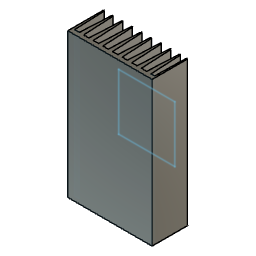
Heat Sink Uncut v1 (Autodesk Fusion 360 design; units mm, degrees)
Autodesk Fusion 360 part; units mm, degrees
sketch "Sketch1" plane through (0, 0, 0) normal (0, 0, 1) x (1, 0, 0)
  line L0 (0, 0) -> (105.15, 0)
  spline S0 degree 5 poles (10.96, 44) (10.99, 44.0758) (11.05, 44.2209) (11.14, 44.4187) (11.26, 44.6419) (11.41, 44.8491) (11.56, 44.9779) (11.71, 45.022) (11.86, 44.9779) (12.01, 44.8491) (12.16, 44.6419) (12.28, 44.4187) (12.37, 44.2209) (12.43, 44.0758) (12.46, 44) knots 0 0 0 0 0 0 0.1 0.2 0.3 0.4 0.5 0.6 0.7 0.8 0.9 1 1 1 1 1 1
  line L1 (10.96, 44) -> (9, 5.4)
  line L2 (12.46, 44) -> (14.42, 5.4)
  spline S1 degree 5 poles (10.96, 44) (10.99, 44.0758) (11.05, 44.2209) (11.14, 44.4187) (11.26, 44.6419) (11.41, 44.8491) (11.56, 44.9779) (11.71, 45.022) (11.86, 44.9779) (12.01, 44.8491) (12.16, 44.6419) (12.28, 44.4187) (12.37, 44.2209) (12.43, 44.0758) (12.46, 44) knots 0 0 0 0 0 0 0.1 0.2 0.3 0.4 0.5 0.6 0.7 0.8 0.9 1 1 1 1 1 1
  line L3 (10.96, 44) -> (9, 5.4)
  line L4 (12.46, 44) -> (14.42, 5.4)
  spline S2 degree 5 poles (10.96, 44) (10.99, 44.0758) (11.05, 44.2209) (11.14, 44.4187) (11.26, 44.6419) (11.41, 44.8491) (11.56, 44.9779) (11.71, 45.022) (11.86, 44.9779) (12.01, 44.8491) (12.16, 44.6419) (12.28, 44.4187) (12.37, 44.2209) (12.43, 44.0758) (12.46, 44) knots 0 0 0 0 0 0 0.1 0.2 0.3 0.4 0.5 0.6 0.7 0.8 0.9 1 1 1 1 1 1
  spline S3 degree 5 poles (10.96, 44) (10.99, 44.0758) (11.05, 44.2209) (11.14, 44.4187) (11.26, 44.6419) (11.41, 44.8491) (11.56, 44.9779) (11.71, 45.022) (11.86, 44.9779) (12.01, 44.8491) (12.16, 44.6419) (12.28, 44.4187) (12.37, 44.2209) (12.43, 44.0758) (12.46, 44) knots 0 0 0 0 0 0 0.1 0.2 0.3 0.4 0.5 0.6 0.7 0.8 0.9 1 1 1 1 1 1
  line L5 (10.96, 44) -> (9, 5.4)
  line L6 (12.46, 44) -> (14.42, 5.4)
  spline S4 degree 5 poles (10.96, 44) (10.99, 44.0758) (11.05, 44.2209) (11.14, 44.4187) (11.26, 44.6419) (11.41, 44.8491) (11.56, 44.9779) (11.71, 45.022) (11.86, 44.9779) (12.01, 44.8491) (12.16, 44.6419) (12.28, 44.4187) (12.37, 44.2209) (12.43, 44.0758) (12.46, 44) knots 0 0 0 0 0 0 0.1 0.2 0.3 0.4 0.5 0.6 0.7 0.8 0.9 1 1 1 1 1 1
  spline S5 degree 5 poles (10.96, 44) (10.99, 44.0758) (11.05, 44.2209) (11.14, 44.4187) (11.26, 44.6419) (11.41, 44.8491) (11.56, 44.9779) (11.71, 45.022) (11.86, 44.9779) (12.01, 44.8491) (12.16, 44.6419) (12.28, 44.4187) (12.37, 44.2209) (12.43, 44.0758) (12.46, 44) knots 0 0 0 0 0 0 0.1 0.2 0.3 0.4 0.5 0.6 0.7 0.8 0.9 1 1 1 1 1 1
  spline S6 degree 5 poles (10.96, 44) (10.99, 44.0758) (11.05, 44.2209) (11.14, 44.4187) (11.26, 44.6419) (11.41, 44.8491) (11.56, 44.9779) (11.71, 45.022) (11.86, 44.9779) (12.01, 44.8491) (12.16, 44.6419) (12.28, 44.4187) (12.37, 44.2209) (12.43, 44.0758) (12.46, 44) knots 0 0 0 0 0 0 0.1 0.2 0.3 0.4 0.5 0.6 0.7 0.8 0.9 1 1 1 1 1 1
  spline S7 degree 5 poles (10.96, 44) (10.99, 44.0758) (11.05, 44.2209) (11.14, 44.4187) (11.26, 44.6419) (11.41, 44.8491) (11.56, 44.9779) (11.71, 45.022) (11.86, 44.9779) (12.01, 44.8491) (12.16, 44.6419) (12.28, 44.4187) (12.37, 44.2209) (12.43, 44.0758) (12.46, 44) knots 0 0 0 0 0 0 0.1 0.2 0.3 0.4 0.5 0.6 0.7 0.8 0.9 1 1 1 1 1 1
  line L7 (10.96, 44) -> (9, 5.4)
  line L8 (12.46, 44) -> (14.42, 5.4)
  spline S8 degree 5 poles (22.96, 44) (22.99, 44.0758) (23.05, 44.2209) (23.14, 44.4187) (23.26, 44.6419) (23.41, 44.8491) (23.56, 44.9779) (23.71, 45.022) (23.86, 44.9779) (24.01, 44.8491) (24.16, 44.6419) (24.28, 44.4187) (24.37, 44.2209) (24.43, 44.0758) (24.46, 44) knots 0 0 0 0 0 0 0.1 0.2 0.3 0.4 0.5 0.6 0.7 0.8 0.9 1 1 1 1 1 1
  spline S9 degree 5 poles (22.96, 44) (22.99, 44.0758) (23.05, 44.2209) (23.14, 44.4187) (23.26, 44.6419) (23.41, 44.8491) (23.56, 44.9779) (23.71, 45.022) (23.86, 44.9779) (24.01, 44.8491) (24.16, 44.6419) (24.28, 44.4187) (24.37, 44.2209) (24.43, 44.0758) (24.46, 44) knots 0 0 0 0 0 0 0.1 0.2 0.3 0.4 0.5 0.6 0.7 0.8 0.9 1 1 1 1 1 1
  spline S10 degree 5 poles (22.96, 44) (22.99, 44.0758) (23.05, 44.2209) (23.14, 44.4187) (23.26, 44.6419) (23.41, 44.8491) (23.56, 44.9779) (23.71, 45.022) (23.86, 44.9779) (24.01, 44.8491) (24.16, 44.6419) (24.28, 44.4187) (24.37, 44.2209) (24.43, 44.0758) (24.46, 44) knots 0 0 0 0 0 0 0.1 0.2 0.3 0.4 0.5 0.6 0.7 0.8 0.9 1 1 1 1 1 1
  spline S11 degree 5 poles (22.96, 44) (22.99, 44.0758) (23.05, 44.2209) (23.14, 44.4187) (23.26, 44.6419) (23.41, 44.8491) (23.56, 44.9779) (23.71, 45.022) (23.86, 44.9779) (24.01, 44.8491) (24.16, 44.6419) (24.28, 44.4187) (24.37, 44.2209) (24.43, 44.0758) (24.46, 44) knots 0 0 0 0 0 0 0.1 0.2 0.3 0.4 0.5 0.6 0.7 0.8 0.9 1 1 1 1 1 1
  spline S12 degree 5 poles (22.96, 44) (22.99, 44.0758) (23.05, 44.2209) (23.14, 44.4187) (23.26, 44.6419) (23.41, 44.8491) (23.56, 44.9779) (23.71, 45.022) (23.86, 44.9779) (24.01, 44.8491) (24.16, 44.6419) (24.28, 44.4187) (24.37, 44.2209) (24.43, 44.0758) (24.46, 44) knots 0 0 0 0 0 0 0.1 0.2 0.3 0.4 0.5 0.6 0.7 0.8 0.9 1 1 1 1 1 1
  spline S13 degree 5 poles (22.96, 44) (22.99, 44.0758) (23.05, 44.2209) (23.14, 44.4187) (23.26, 44.6419) (23.41, 44.8491) (23.56, 44.9779) (23.71, 45.022) (23.86, 44.9779) (24.01, 44.8491) (24.16, 44.6419) (24.28, 44.4187) (24.37, 44.2209) (24.43, 44.0758) (24.46, 44) knots 0 0 0 0 0 0 0.1 0.2 0.3 0.4 0.5 0.6 0.7 0.8 0.9 1 1 1 1 1 1
  spline S14 degree 5 poles (22.96, 44) (22.99, 44.0758) (23.05, 44.2209) (23.14, 44.4187) (23.26, 44.6419) (23.41, 44.8491) (23.56, 44.9779) (23.71, 45.022) (23.86, 44.9779) (24.01, 44.8491) (24.16, 44.6419) (24.28, 44.4187) (24.37, 44.2209) (24.43, 44.0758) (24.46, 44) knots 0 0 0 0 0 0 0.1 0.2 0.3 0.4 0.5 0.6 0.7 0.8 0.9 1 1 1 1 1 1
  spline S15 degree 5 poles (22.96, 44) (22.99, 44.0758) (23.05, 44.2209) (23.14, 44.4187) (23.26, 44.6419) (23.41, 44.8491) (23.56, 44.9779) (23.71, 45.022) (23.86, 44.9779) (24.01, 44.8491) (24.16, 44.6419) (24.28, 44.4187) (24.37, 44.2209) (24.43, 44.0758) (24.46, 44) knots 0 0 0 0 0 0 0.1 0.2 0.3 0.4 0.5 0.6 0.7 0.8 0.9 1 1 1 1 1 1
  line L9 (22.96, 44) -> (21, 5.4)
  line L10 (24.46, 44) -> (26.42, 5.4)
  spline S16 degree 5 poles (34.96, 44) (34.99, 44.0758) (35.05, 44.2209) (35.14, 44.4187) (35.26, 44.6419) (35.41, 44.8491) (35.56, 44.9779) (35.71, 45.022) (35.86, 44.9779) (36.01, 44.8491) (36.16, 44.6419) (36.28, 44.4187) (36.37, 44.2209) (36.43, 44.0758) (36.46, 44) knots 0 0 0 0 0 0 0.1 0.2 0.3 0.4 0.5 0.6 0.7 0.8 0.9 1 1 1 1 1 1
  spline S17 degree 5 poles (34.96, 44) (34.99, 44.0758) (35.05, 44.2209) (35.14, 44.4187) (35.26, 44.6419) (35.41, 44.8491) (35.56, 44.9779) (35.71, 45.022) (35.86, 44.9779) (36.01, 44.8491) (36.16, 44.6419) (36.28, 44.4187) (36.37, 44.2209) (36.43, 44.0758) (36.46, 44) knots 0 0 0 0 0 0 0.1 0.2 0.3 0.4 0.5 0.6 0.7 0.8 0.9 1 1 1 1 1 1
  spline S18 degree 5 poles (34.96, 44) (34.99, 44.0758) (35.05, 44.2209) (35.14, 44.4187) (35.26, 44.6419) (35.41, 44.8491) (35.56, 44.9779) (35.71, 45.022) (35.86, 44.9779) (36.01, 44.8491) (36.16, 44.6419) (36.28, 44.4187) (36.37, 44.2209) (36.43, 44.0758) (36.46, 44) knots 0 0 0 0 0 0 0.1 0.2 0.3 0.4 0.5 0.6 0.7 0.8 0.9 1 1 1 1 1 1
  spline S19 degree 5 poles (34.96, 44) (34.99, 44.0758) (35.05, 44.2209) (35.14, 44.4187) (35.26, 44.6419) (35.41, 44.8491) (35.56, 44.9779) (35.71, 45.022) (35.86, 44.9779) (36.01, 44.8491) (36.16, 44.6419) (36.28, 44.4187) (36.37, 44.2209) (36.43, 44.0758) (36.46, 44) knots 0 0 0 0 0 0 0.1 0.2 0.3 0.4 0.5 0.6 0.7 0.8 0.9 1 1 1 1 1 1
  spline S20 degree 5 poles (34.96, 44) (34.99, 44.0758) (35.05, 44.2209) (35.14, 44.4187) (35.26, 44.6419) (35.41, 44.8491) (35.56, 44.9779) (35.71, 45.022) (35.86, 44.9779) (36.01, 44.8491) (36.16, 44.6419) (36.28, 44.4187) (36.37, 44.2209) (36.43, 44.0758) (36.46, 44) knots 0 0 0 0 0 0 0.1 0.2 0.3 0.4 0.5 0.6 0.7 0.8 0.9 1 1 1 1 1 1
  spline S21 degree 5 poles (34.96, 44) (34.99, 44.0758) (35.05, 44.2209) (35.14, 44.4187) (35.26, 44.6419) (35.41, 44.8491) (35.56, 44.9779) (35.71, 45.022) (35.86, 44.9779) (36.01, 44.8491) (36.16, 44.6419) (36.28, 44.4187) (36.37, 44.2209) (36.43, 44.0758) (36.46, 44) knots 0 0 0 0 0 0 0.1 0.2 0.3 0.4 0.5 0.6 0.7 0.8 0.9 1 1 1 1 1 1
  spline S22 degree 5 poles (34.96, 44) (34.99, 44.0758) (35.05, 44.2209) (35.14, 44.4187) (35.26, 44.6419) (35.41, 44.8491) (35.56, 44.9779) (35.71, 45.022) (35.86, 44.9779) (36.01, 44.8491) (36.16, 44.6419) (36.28, 44.4187) (36.37, 44.2209) (36.43, 44.0758) (36.46, 44) knots 0 0 0 0 0 0 0.1 0.2 0.3 0.4 0.5 0.6 0.7 0.8 0.9 1 1 1 1 1 1
  spline S23 degree 5 poles (34.96, 44) (34.99, 44.0758) (35.05, 44.2209) (35.14, 44.4187) (35.26, 44.6419) (35.41, 44.8491) (35.56, 44.9779) (35.71, 45.022) (35.86, 44.9779) (36.01, 44.8491) (36.16, 44.6419) (36.28, 44.4187) (36.37, 44.2209) (36.43, 44.0758) (36.46, 44) knots 0 0 0 0 0 0 0.1 0.2 0.3 0.4 0.5 0.6 0.7 0.8 0.9 1 1 1 1 1 1
  line L11 (34.96, 44) -> (33, 5.4)
  line L12 (36.46, 44) -> (38.42, 5.4)
  spline S24 degree 5 poles (46.96, 44) (46.99, 44.0758) (47.05, 44.2209) (47.14, 44.4187) (47.26, 44.6419) (47.41, 44.8491) (47.56, 44.9779) (47.71, 45.022) (47.86, 44.9779) (48.01, 44.8491) (48.16, 44.6419) (48.28, 44.4187) (48.37, 44.2209) (48.43, 44.0758) (48.46, 44) knots 0 0 0 0 0 0 0.1 0.2 0.3 0.4 0.5 0.6 0.7 0.8 0.9 1 1 1 1 1 1
  spline S25 degree 5 poles (46.96, 44) (46.99, 44.0758) (47.05, 44.2209) (47.14, 44.4187) (47.26, 44.6419) (47.41, 44.8491) (47.56, 44.9779) (47.71, 45.022) (47.86, 44.9779) (48.01, 44.8491) (48.16, 44.6419) (48.28, 44.4187) (48.37, 44.2209) (48.43, 44.0758) (48.46, 44) knots 0 0 0 0 0 0 0.1 0.2 0.3 0.4 0.5 0.6 0.7 0.8 0.9 1 1 1 1 1 1
  spline S26 degree 5 poles (46.96, 44) (46.99, 44.0758) (47.05, 44.2209) (47.14, 44.4187) (47.26, 44.6419) (47.41, 44.8491) (47.56, 44.9779) (47.71, 45.022) (47.86, 44.9779) (48.01, 44.8491) (48.16, 44.6419) (48.28, 44.4187) (48.37, 44.2209) (48.43, 44.0758) (48.46, 44) knots 0 0 0 0 0 0 0.1 0.2 0.3 0.4 0.5 0.6 0.7 0.8 0.9 1 1 1 1 1 1
  spline S27 degree 5 poles (46.96, 44) (46.99, 44.0758) (47.05, 44.2209) (47.14, 44.4187) (47.26, 44.6419) (47.41, 44.8491) (47.56, 44.9779) (47.71, 45.022) (47.86, 44.9779) (48.01, 44.8491) (48.16, 44.6419) (48.28, 44.4187) (48.37, 44.2209) (48.43, 44.0758) (48.46, 44) knots 0 0 0 0 0 0 0.1 0.2 0.3 0.4 0.5 0.6 0.7 0.8 0.9 1 1 1 1 1 1
  spline S28 degree 5 poles (46.96, 44) (46.99, 44.0758) (47.05, 44.2209) (47.14, 44.4187) (47.26, 44.6419) (47.41, 44.8491) (47.56, 44.9779) (47.71, 45.022) (47.86, 44.9779) (48.01, 44.8491) (48.16, 44.6419) (48.28, 44.4187) (48.37, 44.2209) (48.43, 44.0758) (48.46, 44) knots 0 0 0 0 0 0 0.1 0.2 0.3 0.4 0.5 0.6 0.7 0.8 0.9 1 1 1 1 1 1
  spline S29 degree 5 poles (46.96, 44) (46.99, 44.0758) (47.05, 44.2209) (47.14, 44.4187) (47.26, 44.6419) (47.41, 44.8491) (47.56, 44.9779) (47.71, 45.022) (47.86, 44.9779) (48.01, 44.8491) (48.16, 44.6419) (48.28, 44.4187) (48.37, 44.2209) (48.43, 44.0758) (48.46, 44) knots 0 0 0 0 0 0 0.1 0.2 0.3 0.4 0.5 0.6 0.7 0.8 0.9 1 1 1 1 1 1
  spline S30 degree 5 poles (46.96, 44) (46.99, 44.0758) (47.05, 44.2209) (47.14, 44.4187) (47.26, 44.6419) (47.41, 44.8491) (47.56, 44.9779) (47.71, 45.022) (47.86, 44.9779) (48.01, 44.8491) (48.16, 44.6419) (48.28, 44.4187) (48.37, 44.2209) (48.43, 44.0758) (48.46, 44) knots 0 0 0 0 0 0 0.1 0.2 0.3 0.4 0.5 0.6 0.7 0.8 0.9 1 1 1 1 1 1
  spline S31 degree 5 poles (46.96, 44) (46.99, 44.0758) (47.05, 44.2209) (47.14, 44.4187) (47.26, 44.6419) (47.41, 44.8491) (47.56, 44.9779) (47.71, 45.022) (47.86, 44.9779) (48.01, 44.8491) (48.16, 44.6419) (48.28, 44.4187) (48.37, 44.2209) (48.43, 44.0758) (48.46, 44) knots 0 0 0 0 0 0 0.1 0.2 0.3 0.4 0.5 0.6 0.7 0.8 0.9 1 1 1 1 1 1
  line L13 (46.96, 44) -> (45, 5.4)
  line L14 (48.46, 44) -> (50.42, 5.4)
  spline S32 degree 5 poles (58.96, 44) (58.99, 44.0758) (59.05, 44.2209) (59.14, 44.4187) (59.26, 44.6419) (59.41, 44.8491) (59.56, 44.9779) (59.71, 45.022) (59.86, 44.9779) (60.01, 44.8491) (60.16, 44.6419) (60.28, 44.4187) (60.37, 44.2209) (60.43, 44.0758) (60.46, 44) knots 0 0 0 0 0 0 0.1 0.2 0.3 0.4 0.5 0.6 0.7 0.8 0.9 1 1 1 1 1 1
  spline S33 degree 5 poles (58.96, 44) (58.99, 44.0758) (59.05, 44.2209) (59.14, 44.4187) (59.26, 44.6419) (59.41, 44.8491) (59.56, 44.9779) (59.71, 45.022) (59.86, 44.9779) (60.01, 44.8491) (60.16, 44.6419) (60.28, 44.4187) (60.37, 44.2209) (60.43, 44.0758) (60.46, 44) knots 0 0 0 0 0 0 0.1 0.2 0.3 0.4 0.5 0.6 0.7 0.8 0.9 1 1 1 1 1 1
  spline S34 degree 5 poles (58.96, 44) (58.99, 44.0758) (59.05, 44.2209) (59.14, 44.4187) (59.26, 44.6419) (59.41, 44.8491) (59.56, 44.9779) (59.71, 45.022) (59.86, 44.9779) (60.01, 44.8491) (60.16, 44.6419) (60.28, 44.4187) (60.37, 44.2209) (60.43, 44.0758) (60.46, 44) knots 0 0 0 0 0 0 0.1 0.2 0.3 0.4 0.5 0.6 0.7 0.8 0.9 1 1 1 1 1 1
  spline S35 degree 5 poles (58.96, 44) (58.99, 44.0758) (59.05, 44.2209) (59.14, 44.4187) (59.26, 44.6419) (59.41, 44.8491) (59.56, 44.9779) (59.71, 45.022) (59.86, 44.9779) (60.01, 44.8491) (60.16, 44.6419) (60.28, 44.4187) (60.37, 44.2209) (60.43, 44.0758) (60.46, 44) knots 0 0 0 0 0 0 0.1 0.2 0.3 0.4 0.5 0.6 0.7 0.8 0.9 1 1 1 1 1 1
  spline S36 degree 5 poles (58.96, 44) (58.99, 44.0758) (59.05, 44.2209) (59.14, 44.4187) (59.26, 44.6419) (59.41, 44.8491) (59.56, 44.9779) (59.71, 45.022) (59.86, 44.9779) (60.01, 44.8491) (60.16, 44.6419) (60.28, 44.4187) (60.37, 44.2209) (60.43, 44.0758) (60.46, 44) knots 0 0 0 0 0 0 0.1 0.2 0.3 0.4 0.5 0.6 0.7 0.8 0.9 1 1 1 1 1 1
  spline S37 degree 5 poles (58.96, 44) (58.99, 44.0758) (59.05, 44.2209) (59.14, 44.4187) (59.26, 44.6419) (59.41, 44.8491) (59.56, 44.9779) (59.71, 45.022) (59.86, 44.9779) (60.01, 44.8491) (60.16, 44.6419) (60.28, 44.4187) (60.37, 44.2209) (60.43, 44.0758) (60.46, 44) knots 0 0 0 0 0 0 0.1 0.2 0.3 0.4 0.5 0.6 0.7 0.8 0.9 1 1 1 1 1 1
  spline S38 degree 5 poles (58.96, 44) (58.99, 44.0758) (59.05, 44.2209) (59.14, 44.4187) (59.26, 44.6419) (59.41, 44.8491) (59.56, 44.9779) (59.71, 45.022) (59.86, 44.9779) (60.01, 44.8491) (60.16, 44.6419) (60.28, 44.4187) (60.37, 44.2209) (60.43, 44.0758) (60.46, 44) knots 0 0 0 0 0 0 0.1 0.2 0.3 0.4 0.5 0.6 0.7 0.8 0.9 1 1 1 1 1 1
  spline S39 degree 5 poles (58.96, 44) (58.99, 44.0758) (59.05, 44.2209) (59.14, 44.4187) (59.26, 44.6419) (59.41, 44.8491) (59.56, 44.9779) (59.71, 45.022) (59.86, 44.9779) (60.01, 44.8491) (60.16, 44.6419) (60.28, 44.4187) (60.37, 44.2209) (60.43, 44.0758) (60.46, 44) knots 0 0 0 0 0 0 0.1 0.2 0.3 0.4 0.5 0.6 0.7 0.8 0.9 1 1 1 1 1 1
  line L15 (58.96, 44) -> (57, 5.4)
  line L16 (60.46, 44) -> (62.42, 5.4)
  spline S40 degree 5 poles (58.96, 44) (58.99, 44.0758) (59.05, 44.2209) (59.14, 44.4187) (59.26, 44.6419) (59.41, 44.8491) (59.56, 44.9779) (59.71, 45.022) (59.86, 44.9779) (60.01, 44.8491) (60.16, 44.6419) (60.28, 44.4187) (60.37, 44.2209) (60.43, 44.0758) (60.46, 44) knots 0 0 0 0 0 0 0.1 0.2 0.3 0.4 0.5 0.6 0.7 0.8 0.9 1 1 1 1 1 1
  spline S41 degree 5 poles (58.96, 44) (58.99, 44.0758) (59.05, 44.2209) (59.14, 44.4187) (59.26, 44.6419) (59.41, 44.8491) (59.56, 44.9779) (59.71, 45.022) (59.86, 44.9779) (60.01, 44.8491) (60.16, 44.6419) (60.28, 44.4187) (60.37, 44.2209) (60.43, 44.0758) (60.46, 44) knots 0 0 0 0 0 0 0.1 0.2 0.3 0.4 0.5 0.6 0.7 0.8 0.9 1 1 1 1 1 1
  spline S42 degree 5 poles (58.96, 44) (58.99, 44.0758) (59.05, 44.2209) (59.14, 44.4187) (59.26, 44.6419) (59.41, 44.8491) (59.56, 44.9779) (59.71, 45.022) (59.86, 44.9779) (60.01, 44.8491) (60.16, 44.6419) (60.28, 44.4187) (60.37, 44.2209) (60.43, 44.0758) (60.46, 44) knots 0 0 0 0 0 0 0.1 0.2 0.3 0.4 0.5 0.6 0.7 0.8 0.9 1 1 1 1 1 1
  spline S43 degree 5 poles (58.96, 44) (58.99, 44.0758) (59.05, 44.2209) (59.14, 44.4187) (59.26, 44.6419) (59.41, 44.8491) (59.56, 44.9779) (59.71, 45.022) (59.86, 44.9779) (60.01, 44.8491) (60.16, 44.6419) (60.28, 44.4187) (60.37, 44.2209) (60.43, 44.0758) (60.46, 44) knots 0 0 0 0 0 0 0.1 0.2 0.3 0.4 0.5 0.6 0.7 0.8 0.9 1 1 1 1 1 1
  spline S44 degree 5 poles (58.96, 44) (58.99, 44.0758) (59.05, 44.2209) (59.14, 44.4187) (59.26, 44.6419) (59.41, 44.8491) (59.56, 44.9779) (59.71, 45.022) (59.86, 44.9779) (60.01, 44.8491) (60.16, 44.6419) (60.28, 44.4187) (60.37, 44.2209) (60.43, 44.0758) (60.46, 44) knots 0 0 0 0 0 0 0.1 0.2 0.3 0.4 0.5 0.6 0.7 0.8 0.9 1 1 1 1 1 1
  spline S45 degree 5 poles (58.96, 44) (58.99, 44.0758) (59.05, 44.2209) (59.14, 44.4187) (59.26, 44.6419) (59.41, 44.8491) (59.56, 44.9779) (59.71, 45.022) (59.86, 44.9779) (60.01, 44.8491) (60.16, 44.6419) (60.28, 44.4187) (60.37, 44.2209) (60.43, 44.0758) (60.46, 44) knots 0 0 0 0 0 0 0.1 0.2 0.3 0.4 0.5 0.6 0.7 0.8 0.9 1 1 1 1 1 1
  spline S46 degree 5 poles (58.96, 44) (58.99, 44.0758) (59.05, 44.2209) (59.14, 44.4187) (59.26, 44.6419) (59.41, 44.8491) (59.56, 44.9779) (59.71, 45.022) (59.86, 44.9779) (60.01, 44.8491) (60.16, 44.6419) (60.28, 44.4187) (60.37, 44.2209) (60.43, 44.0758) (60.46, 44) knots 0 0 0 0 0 0 0.1 0.2 0.3 0.4 0.5 0.6 0.7 0.8 0.9 1 1 1 1 1 1
  spline S47 degree 5 poles (58.96, 44) (58.99, 44.0758) (59.05, 44.2209) (59.14, 44.4187) (59.26, 44.6419) (59.41, 44.8491) (59.56, 44.9779) (59.71, 45.022) (59.86, 44.9779) (60.01, 44.8491) (60.16, 44.6419) (60.28, 44.4187) (60.37, 44.2209) (60.43, 44.0758) (60.46, 44) knots 0 0 0 0 0 0 0.1 0.2 0.3 0.4 0.5 0.6 0.7 0.8 0.9 1 1 1 1 1 1
  spline S48 degree 5 poles (70.96, 44) (70.99, 44.0758) (71.05, 44.2209) (71.14, 44.4187) (71.26, 44.6419) (71.41, 44.8491) (71.56, 44.9779) (71.71, 45.022) (71.86, 44.9779) (72.01, 44.8491) (72.16, 44.6419) (72.28, 44.4187) (72.37, 44.2209) (72.43, 44.0758) (72.46, 44) knots 0 0 0 0 0 0 0.1 0.2 0.3 0.4 0.5 0.6 0.7 0.8 0.9 1 1 1 1 1 1
  spline S49 degree 5 poles (70.96, 44) (70.99, 44.0758) (71.05, 44.2209) (71.14, 44.4187) (71.26, 44.6419) (71.41, 44.8491) (71.56, 44.9779) (71.71, 45.022) (71.86, 44.9779) (72.01, 44.8491) (72.16, 44.6419) (72.28, 44.4187) (72.37, 44.2209) (72.43, 44.0758) (72.46, 44) knots 0 0 0 0 0 0 0.1 0.2 0.3 0.4 0.5 0.6 0.7 0.8 0.9 1 1 1 1 1 1
  spline S50 degree 5 poles (70.96, 44) (70.99, 44.0758) (71.05, 44.2209) (71.14, 44.4187) (71.26, 44.6419) (71.41, 44.8491) (71.56, 44.9779) (71.71, 45.022) (71.86, 44.9779) (72.01, 44.8491) (72.16, 44.6419) (72.28, 44.4187) (72.37, 44.2209) (72.43, 44.0758) (72.46, 44) knots 0 0 0 0 0 0 0.1 0.2 0.3 0.4 0.5 0.6 0.7 0.8 0.9 1 1 1 1 1 1
  spline S51 degree 5 poles (70.96, 44) (70.99, 44.0758) (71.05, 44.2209) (71.14, 44.4187) (71.26, 44.6419) (71.41, 44.8491) (71.56, 44.9779) (71.71, 45.022) (71.86, 44.9779) (72.01, 44.8491) (72.16, 44.6419) (72.28, 44.4187) (72.37, 44.2209) (72.43, 44.0758) (72.46, 44) knots 0 0 0 0 0 0 0.1 0.2 0.3 0.4 0.5 0.6 0.7 0.8 0.9 1 1 1 1 1 1
  spline S52 degree 5 poles (70.96, 44) (70.99, 44.0758) (71.05, 44.2209) (71.14, 44.4187) (71.26, 44.6419) (71.41, 44.8491) (71.56, 44.9779) (71.71, 45.022) (71.86, 44.9779) (72.01, 44.8491) (72.16, 44.6419) (72.28, 44.4187) (72.37, 44.2209) (72.43, 44.0758) (72.46, 44) knots 0 0 0 0 0 0 0.1 0.2 0.3 0.4 0.5 0.6 0.7 0.8 0.9 1 1 1 1 1 1
  spline S53 degree 5 poles (70.96, 44) (70.99, 44.0758) (71.05, 44.2209) (71.14, 44.4187) (71.26, 44.6419) (71.41, 44.8491) (71.56, 44.9779) (71.71, 45.022) (71.86, 44.9779) (72.01, 44.8491) (72.16, 44.6419) (72.28, 44.4187) (72.37, 44.2209) (72.43, 44.0758) (72.46, 44) knots 0 0 0 0 0 0 0.1 0.2 0.3 0.4 0.5 0.6 0.7 0.8 0.9 1 1 1 1 1 1
  spline S54 degree 5 poles (70.96, 44) (70.99, 44.0758) (71.05, 44.2209) (71.14, 44.4187) (71.26, 44.6419) (71.41, 44.8491) (71.56, 44.9779) (71.71, 45.022) (71.86, 44.9779) (72.01, 44.8491) (72.16, 44.6419) (72.28, 44.4187) (72.37, 44.2209) (72.43, 44.0758) (72.46, 44) knots 0 0 0 0 0 0 0.1 0.2 0.3 0.4 0.5 0.6 0.7 0.8 0.9 1 1 1 1 1 1
  spline S55 degree 5 poles (70.96, 44) (70.99, 44.0758) (71.05, 44.2209) (71.14, 44.4187) (71.26, 44.6419) (71.41, 44.8491) (71.56, 44.9779) (71.71, 45.022) (71.86, 44.9779) (72.01, 44.8491) (72.16, 44.6419) (72.28, 44.4187) (72.37, 44.2209) (72.43, 44.0758) (72.46, 44) knots 0 0 0 0 0 0 0.1 0.2 0.3 0.4 0.5 0.6 0.7 0.8 0.9 1 1 1 1 1 1
  spline S56 degree 5 poles (70.96, 44) (70.99, 44.0758) (71.05, 44.2209) (71.14, 44.4187) (71.26, 44.6419) (71.41, 44.8491) (71.56, 44.9779) (71.71, 45.022) (71.86, 44.9779) (72.01, 44.8491) (72.16, 44.6419) (72.28, 44.4187) (72.37, 44.2209) (72.43, 44.0758) (72.46, 44) knots 0 0 0 0 0 0 0.1 0.2 0.3 0.4 0.5 0.6 0.7 0.8 0.9 1 1 1 1 1 1
  spline S57 degree 5 poles (70.96, 44) (70.99, 44.0758) (71.05, 44.2209) (71.14, 44.4187) (71.26, 44.6419) (71.41, 44.8491) (71.56, 44.9779) (71.71, 45.022) (71.86, 44.9779) (72.01, 44.8491) (72.16, 44.6419) (72.28, 44.4187) (72.37, 44.2209) (72.43, 44.0758) (72.46, 44) knots 0 0 0 0 0 0 0.1 0.2 0.3 0.4 0.5 0.6 0.7 0.8 0.9 1 1 1 1 1 1
  spline S58 degree 5 poles (70.96, 44) (70.99, 44.0758) (71.05, 44.2209) (71.14, 44.4187) (71.26, 44.6419) (71.41, 44.8491) (71.56, 44.9779) (71.71, 45.022) (71.86, 44.9779) (72.01, 44.8491) (72.16, 44.6419) (72.28, 44.4187) (72.37, 44.2209) (72.43, 44.0758) (72.46, 44) knots 0 0 0 0 0 0 0.1 0.2 0.3 0.4 0.5 0.6 0.7 0.8 0.9 1 1 1 1 1 1
  spline S59 degree 5 poles (70.96, 44) (70.99, 44.0758) (71.05, 44.2209) (71.14, 44.4187) (71.26, 44.6419) (71.41, 44.8491) (71.56, 44.9779) (71.71, 45.022) (71.86, 44.9779) (72.01, 44.8491) (72.16, 44.6419) (72.28, 44.4187) (72.37, 44.2209) (72.43, 44.0758) (72.46, 44) knots 0 0 0 0 0 0 0.1 0.2 0.3 0.4 0.5 0.6 0.7 0.8 0.9 1 1 1 1 1 1
  spline S60 degree 5 poles (70.96, 44) (70.99, 44.0758) (71.05, 44.2209) (71.14, 44.4187) (71.26, 44.6419) (71.41, 44.8491) (71.56, 44.9779) (71.71, 45.022) (71.86, 44.9779) (72.01, 44.8491) (72.16, 44.6419) (72.28, 44.4187) (72.37, 44.2209) (72.43, 44.0758) (72.46, 44) knots 0 0 0 0 0 0 0.1 0.2 0.3 0.4 0.5 0.6 0.7 0.8 0.9 1 1 1 1 1 1
  spline S61 degree 5 poles (70.96, 44) (70.99, 44.0758) (71.05, 44.2209) (71.14, 44.4187) (71.26, 44.6419) (71.41, 44.8491) (71.56, 44.9779) (71.71, 45.022) (71.86, 44.9779) (72.01, 44.8491) (72.16, 44.6419) (72.28, 44.4187) (72.37, 44.2209) (72.43, 44.0758) (72.46, 44) knots 0 0 0 0 0 0 0.1 0.2 0.3 0.4 0.5 0.6 0.7 0.8 0.9 1 1 1 1 1 1
  spline S62 degree 5 poles (70.96, 44) (70.99, 44.0758) (71.05, 44.2209) (71.14, 44.4187) (71.26, 44.6419) (71.41, 44.8491) (71.56, 44.9779) (71.71, 45.022) (71.86, 44.9779) (72.01, 44.8491) (72.16, 44.6419) (72.28, 44.4187) (72.37, 44.2209) (72.43, 44.0758) (72.46, 44) knots 0 0 0 0 0 0 0.1 0.2 0.3 0.4 0.5 0.6 0.7 0.8 0.9 1 1 1 1 1 1
  spline S63 degree 5 poles (70.96, 44) (70.99, 44.0758) (71.05, 44.2209) (71.14, 44.4187) (71.26, 44.6419) (71.41, 44.8491) (71.56, 44.9779) (71.71, 45.022) (71.86, 44.9779) (72.01, 44.8491) (72.16, 44.6419) (72.28, 44.4187) (72.37, 44.2209) (72.43, 44.0758) (72.46, 44) knots 0 0 0 0 0 0 0.1 0.2 0.3 0.4 0.5 0.6 0.7 0.8 0.9 1 1 1 1 1 1
  line L17 (70.96, 44) -> (69, 5.4)
  line L18 (72.46, 44) -> (74.42, 5.4)
  spline S64 degree 5 poles (82.96, 44) (82.99, 44.0758) (83.05, 44.2209) (83.14, 44.4187) (83.26, 44.6419) (83.41, 44.8491) (83.56, 44.9779) (83.71, 45.022) (83.86, 44.9779) (84.01, 44.8491) (84.16, 44.6419) (84.28, 44.4187) (84.37, 44.2209) (84.43, 44.0758) (84.46, 44) knots 0 0 0 0 0 0 0.1 0.2 0.3 0.4 0.5 0.6 0.7 0.8 0.9 1 1 1 1 1 1
  spline S65 degree 5 poles (82.96, 44) (82.99, 44.0758) (83.05, 44.2209) (83.14, 44.4187) (83.26, 44.6419) (83.41, 44.8491) (83.56, 44.9779) (83.71, 45.022) (83.86, 44.9779) (84.01, 44.8491) (84.16, 44.6419) (84.28, 44.4187) (84.37, 44.2209) (84.43, 44.0758) (84.46, 44) knots 0 0 0 0 0 0 0.1 0.2 0.3 0.4 0.5 0.6 0.7 0.8 0.9 1 1 1 1 1 1
  spline S66 degree 5 poles (82.96, 44) (82.99, 44.0758) (83.05, 44.2209) (83.14, 44.4187) (83.26, 44.6419) (83.41, 44.8491) (83.56, 44.9779) (83.71, 45.022) (83.86, 44.9779) (84.01, 44.8491) (84.16, 44.6419) (84.28, 44.4187) (84.37, 44.2209) (84.43, 44.0758) (84.46, 44) knots 0 0 0 0 0 0 0.1 0.2 0.3 0.4 0.5 0.6 0.7 0.8 0.9 1 1 1 1 1 1
  spline S67 degree 5 poles (82.96, 44) (82.99, 44.0758) (83.05, 44.2209) (83.14, 44.4187) (83.26, 44.6419) (83.41, 44.8491) (83.56, 44.9779) (83.71, 45.022) (83.86, 44.9779) (84.01, 44.8491) (84.16, 44.6419) (84.28, 44.4187) (84.37, 44.2209) (84.43, 44.0758) (84.46, 44) knots 0 0 0 0 0 0 0.1 0.2 0.3 0.4 0.5 0.6 0.7 0.8 0.9 1 1 1 1 1 1
  spline S68 degree 5 poles (82.96, 44) (82.99, 44.0758) (83.05, 44.2209) (83.14, 44.4187) (83.26, 44.6419) (83.41, 44.8491) (83.56, 44.9779) (83.71, 45.022) (83.86, 44.9779) (84.01, 44.8491) (84.16, 44.6419) (84.28, 44.4187) (84.37, 44.2209) (84.43, 44.0758) (84.46, 44) knots 0 0 0 0 0 0 0.1 0.2 0.3 0.4 0.5 0.6 0.7 0.8 0.9 1 1 1 1 1 1
  spline S69 degree 5 poles (82.96, 44) (82.99, 44.0758) (83.05, 44.2209) (83.14, 44.4187) (83.26, 44.6419) (83.41, 44.8491) (83.56, 44.9779) (83.71, 45.022) (83.86, 44.9779) (84.01, 44.8491) (84.16, 44.6419) (84.28, 44.4187) (84.37, 44.2209) (84.43, 44.0758) (84.46, 44) knots 0 0 0 0 0 0 0.1 0.2 0.3 0.4 0.5 0.6 0.7 0.8 0.9 1 1 1 1 1 1
  spline S70 degree 5 poles (82.96, 44) (82.99, 44.0758) (83.05, 44.2209) (83.14, 44.4187) (83.26, 44.6419) (83.41, 44.8491) (83.56, 44.9779) (83.71, 45.022) (83.86, 44.9779) (84.01, 44.8491) (84.16, 44.6419) (84.28, 44.4187) (84.37, 44.2209) (84.43, 44.0758) (84.46, 44) knots 0 0 0 0 0 0 0.1 0.2 0.3 0.4 0.5 0.6 0.7 0.8 0.9 1 1 1 1 1 1
  spline S71 degree 5 poles (82.96, 44) (82.99, 44.0758) (83.05, 44.2209) (83.14, 44.4187) (83.26, 44.6419) (83.41, 44.8491) (83.56, 44.9779) (83.71, 45.022) (83.86, 44.9779) (84.01, 44.8491) (84.16, 44.6419) (84.28, 44.4187) (84.37, 44.2209) (84.43, 44.0758) (84.46, 44) knots 0 0 0 0 0 0 0.1 0.2 0.3 0.4 0.5 0.6 0.7 0.8 0.9 1 1 1 1 1 1
  spline S72 degree 5 poles (82.96, 44) (82.99, 44.0758) (83.05, 44.2209) (83.14, 44.4187) (83.26, 44.6419) (83.41, 44.8491) (83.56, 44.9779) (83.71, 45.022) (83.86, 44.9779) (84.01, 44.8491) (84.16, 44.6419) (84.28, 44.4187) (84.37, 44.2209) (84.43, 44.0758) (84.46, 44) knots 0 0 0 0 0 0 0.1 0.2 0.3 0.4 0.5 0.6 0.7 0.8 0.9 1 1 1 1 1 1
  spline S73 degree 5 poles (82.96, 44) (82.99, 44.0758) (83.05, 44.2209) (83.14, 44.4187) (83.26, 44.6419) (83.41, 44.8491) (83.56, 44.9779) (83.71, 45.022) (83.86, 44.9779) (84.01, 44.8491) (84.16, 44.6419) (84.28, 44.4187) (84.37, 44.2209) (84.43, 44.0758) (84.46, 44) knots 0 0 0 0 0 0 0.1 0.2 0.3 0.4 0.5 0.6 0.7 0.8 0.9 1 1 1 1 1 1
  spline S74 degree 5 poles (82.96, 44) (82.99, 44.0758) (83.05, 44.2209) (83.14, 44.4187) (83.26, 44.6419) (83.41, 44.8491) (83.56, 44.9779) (83.71, 45.022) (83.86, 44.9779) (84.01, 44.8491) (84.16, 44.6419) (84.28, 44.4187) (84.37, 44.2209) (84.43, 44.0758) (84.46, 44) knots 0 0 0 0 0 0 0.1 0.2 0.3 0.4 0.5 0.6 0.7 0.8 0.9 1 1 1 1 1 1
  spline S75 degree 5 poles (82.96, 44) (82.99, 44.0758) (83.05, 44.2209) (83.14, 44.4187) (83.26, 44.6419) (83.41, 44.8491) (83.56, 44.9779) (83.71, 45.022) (83.86, 44.9779) (84.01, 44.8491) (84.16, 44.6419) (84.28, 44.4187) (84.37, 44.2209) (84.43, 44.0758) (84.46, 44) knots 0 0 0 0 0 0 0.1 0.2 0.3 0.4 0.5 0.6 0.7 0.8 0.9 1 1 1 1 1 1
  spline S76 degree 5 poles (82.96, 44) (82.99, 44.0758) (83.05, 44.2209) (83.14, 44.4187) (83.26, 44.6419) (83.41, 44.8491) (83.56, 44.9779) (83.71, 45.022) (83.86, 44.9779) (84.01, 44.8491) (84.16, 44.6419) (84.28, 44.4187) (84.37, 44.2209) (84.43, 44.0758) (84.46, 44) knots 0 0 0 0 0 0 0.1 0.2 0.3 0.4 0.5 0.6 0.7 0.8 0.9 1 1 1 1 1 1
  spline S77 degree 5 poles (82.96, 44) (82.99, 44.0758) (83.05, 44.2209) (83.14, 44.4187) (83.26, 44.6419) (83.41, 44.8491) (83.56, 44.9779) (83.71, 45.022) (83.86, 44.9779) (84.01, 44.8491) (84.16, 44.6419) (84.28, 44.4187) (84.37, 44.2209) (84.43, 44.0758) (84.46, 44) knots 0 0 0 0 0 0 0.1 0.2 0.3 0.4 0.5 0.6 0.7 0.8 0.9 1 1 1 1 1 1
  spline S78 degree 5 poles (82.96, 44) (82.99, 44.0758) (83.05, 44.2209) (83.14, 44.4187) (83.26, 44.6419) (83.41, 44.8491) (83.56, 44.9779) (83.71, 45.022) (83.86, 44.9779) (84.01, 44.8491) (84.16, 44.6419) (84.28, 44.4187) (84.37, 44.2209) (84.43, 44.0758) (84.46, 44) knots 0 0 0 0 0 0 0.1 0.2 0.3 0.4 0.5 0.6 0.7 0.8 0.9 1 1 1 1 1 1
  spline S79 degree 5 poles (82.96, 44) (82.99, 44.0758) (83.05, 44.2209) (83.14, 44.4187) (83.26, 44.6419) (83.41, 44.8491) (83.56, 44.9779) (83.71, 45.022) (83.86, 44.9779) (84.01, 44.8491) (84.16, 44.6419) (84.28, 44.4187) (84.37, 44.2209) (84.43, 44.0758) (84.46, 44) knots 0 0 0 0 0 0 0.1 0.2 0.3 0.4 0.5 0.6 0.7 0.8 0.9 1 1 1 1 1 1
  line L19 (82.96, 44) -> (81, 5.4)
  line L20 (84.46, 44) -> (86.42, 5.4)
  spline S80 degree 5 poles (94.96, 44) (94.99, 44.0758) (95.05, 44.2209) (95.14, 44.4187) (95.26, 44.6419) (95.41, 44.8491) (95.56, 44.9779) (95.71, 45.022) (95.86, 44.9779) (96.01, 44.8491) (96.16, 44.6419) (96.28, 44.4187) (96.37, 44.2209) (96.43, 44.0758) (96.46, 44) knots 0 0 0 0 0 0 0.1 0.2 0.3 0.4 0.5 0.6 0.7 0.8 0.9 1 1 1 1 1 1
  spline S81 degree 5 poles (94.96, 44) (94.99, 44.0758) (95.05, 44.2209) (95.14, 44.4187) (95.26, 44.6419) (95.41, 44.8491) (95.56, 44.9779) (95.71, 45.022) (95.86, 44.9779) (96.01, 44.8491) (96.16, 44.6419) (96.28, 44.4187) (96.37, 44.2209) (96.43, 44.0758) (96.46, 44) knots 0 0 0 0 0 0 0.1 0.2 0.3 0.4 0.5 0.6 0.7 0.8 0.9 1 1 1 1 1 1
  spline S82 degree 5 poles (94.96, 44) (94.99, 44.0758) (95.05, 44.2209) (95.14, 44.4187) (95.26, 44.6419) (95.41, 44.8491) (95.56, 44.9779) (95.71, 45.022) (95.86, 44.9779) (96.01, 44.8491) (96.16, 44.6419) (96.28, 44.4187) (96.37, 44.2209) (96.43, 44.0758) (96.46, 44) knots 0 0 0 0 0 0 0.1 0.2 0.3 0.4 0.5 0.6 0.7 0.8 0.9 1 1 1 1 1 1
  spline S83 degree 5 poles (94.96, 44) (94.99, 44.0758) (95.05, 44.2209) (95.14, 44.4187) (95.26, 44.6419) (95.41, 44.8491) (95.56, 44.9779) (95.71, 45.022) (95.86, 44.9779) (96.01, 44.8491) (96.16, 44.6419) (96.28, 44.4187) (96.37, 44.2209) (96.43, 44.0758) (96.46, 44) knots 0 0 0 0 0 0 0.1 0.2 0.3 0.4 0.5 0.6 0.7 0.8 0.9 1 1 1 1 1 1
  spline S84 degree 5 poles (94.96, 44) (94.99, 44.0758) (95.05, 44.2209) (95.14, 44.4187) (95.26, 44.6419) (95.41, 44.8491) (95.56, 44.9779) (95.71, 45.022) (95.86, 44.9779) (96.01, 44.8491) (96.16, 44.6419) (96.28, 44.4187) (96.37, 44.2209) (96.43, 44.0758) (96.46, 44) knots 0 0 0 0 0 0 0.1 0.2 0.3 0.4 0.5 0.6 0.7 0.8 0.9 1 1 1 1 1 1
  spline S85 degree 5 poles (94.96, 44) (94.99, 44.0758) (95.05, 44.2209) (95.14, 44.4187) (95.26, 44.6419) (95.41, 44.8491) (95.56, 44.9779) (95.71, 45.022) (95.86, 44.9779) (96.01, 44.8491) (96.16, 44.6419) (96.28, 44.4187) (96.37, 44.2209) (96.43, 44.0758) (96.46, 44) knots 0 0 0 0 0 0 0.1 0.2 0.3 0.4 0.5 0.6 0.7 0.8 0.9 1 1 1 1 1 1
  spline S86 degree 5 poles (94.96, 44) (94.99, 44.0758) (95.05, 44.2209) (95.14, 44.4187) (95.26, 44.6419) (95.41, 44.8491) (95.56, 44.9779) (95.71, 45.022) (95.86, 44.9779) (96.01, 44.8491) (96.16, 44.6419) (96.28, 44.4187) (96.37, 44.2209) (96.43, 44.0758) (96.46, 44) knots 0 0 0 0 0 0 0.1 0.2 0.3 0.4 0.5 0.6 0.7 0.8 0.9 1 1 1 1 1 1
  spline S87 degree 5 poles (94.96, 44) (94.99, 44.0758) (95.05, 44.2209) (95.14, 44.4187) (95.26, 44.6419) (95.41, 44.8491) (95.56, 44.9779) (95.71, 45.022) (95.86, 44.9779) (96.01, 44.8491) (96.16, 44.6419) (96.28, 44.4187) (96.37, 44.2209) (96.43, 44.0758) (96.46, 44) knots 0 0 0 0 0 0 0.1 0.2 0.3 0.4 0.5 0.6 0.7 0.8 0.9 1 1 1 1 1 1
  spline S88 degree 5 poles (94.96, 44) (94.99, 44.0758) (95.05, 44.2209) (95.14, 44.4187) (95.26, 44.6419) (95.41, 44.8491) (95.56, 44.9779) (95.71, 45.022) (95.86, 44.9779) (96.01, 44.8491) (96.16, 44.6419) (96.28, 44.4187) (96.37, 44.2209) (96.43, 44.0758) (96.46, 44) knots 0 0 0 0 0 0 0.1 0.2 0.3 0.4 0.5 0.6 0.7 0.8 0.9 1 1 1 1 1 1
  spline S89 degree 5 poles (94.96, 44) (94.99, 44.0758) (95.05, 44.2209) (95.14, 44.4187) (95.26, 44.6419) (95.41, 44.8491) (95.56, 44.9779) (95.71, 45.022) (95.86, 44.9779) (96.01, 44.8491) (96.16, 44.6419) (96.28, 44.4187) (96.37, 44.2209) (96.43, 44.0758) (96.46, 44) knots 0 0 0 0 0 0 0.1 0.2 0.3 0.4 0.5 0.6 0.7 0.8 0.9 1 1 1 1 1 1
  spline S90 degree 5 poles (94.96, 44) (94.99, 44.0758) (95.05, 44.2209) (95.14, 44.4187) (95.26, 44.6419) (95.41, 44.8491) (95.56, 44.9779) (95.71, 45.022) (95.86, 44.9779) (96.01, 44.8491) (96.16, 44.6419) (96.28, 44.4187) (96.37, 44.2209) (96.43, 44.0758) (96.46, 44) knots 0 0 0 0 0 0 0.1 0.2 0.3 0.4 0.5 0.6 0.7 0.8 0.9 1 1 1 1 1 1
  spline S91 degree 5 poles (94.96, 44) (94.99, 44.0758) (95.05, 44.2209) (95.14, 44.4187) (95.26, 44.6419) (95.41, 44.8491) (95.56, 44.9779) (95.71, 45.022) (95.86, 44.9779) (96.01, 44.8491) (96.16, 44.6419) (96.28, 44.4187) (96.37, 44.2209) (96.43, 44.0758) (96.46, 44) knots 0 0 0 0 0 0 0.1 0.2 0.3 0.4 0.5 0.6 0.7 0.8 0.9 1 1 1 1 1 1
  spline S92 degree 5 poles (94.96, 44) (94.99, 44.0758) (95.05, 44.2209) (95.14, 44.4187) (95.26, 44.6419) (95.41, 44.8491) (95.56, 44.9779) (95.71, 45.022) (95.86, 44.9779) (96.01, 44.8491) (96.16, 44.6419) (96.28, 44.4187) (96.37, 44.2209) (96.43, 44.0758) (96.46, 44) knots 0 0 0 0 0 0 0.1 0.2 0.3 0.4 0.5 0.6 0.7 0.8 0.9 1 1 1 1 1 1
  spline S93 degree 5 poles (94.96, 44) (94.99, 44.0758) (95.05, 44.2209) (95.14, 44.4187) (95.26, 44.6419) (95.41, 44.8491) (95.56, 44.9779) (95.71, 45.022) (95.86, 44.9779) (96.01, 44.8491) (96.16, 44.6419) (96.28, 44.4187) (96.37, 44.2209) (96.43, 44.0758) (96.46, 44) knots 0 0 0 0 0 0 0.1 0.2 0.3 0.4 0.5 0.6 0.7 0.8 0.9 1 1 1 1 1 1
  spline S94 degree 5 poles (94.96, 44) (94.99, 44.0758) (95.05, 44.2209) (95.14, 44.4187) (95.26, 44.6419) (95.41, 44.8491) (95.56, 44.9779) (95.71, 45.022) (95.86, 44.9779) (96.01, 44.8491) (96.16, 44.6419) (96.28, 44.4187) (96.37, 44.2209) (96.43, 44.0758) (96.46, 44) knots 0 0 0 0 0 0 0.1 0.2 0.3 0.4 0.5 0.6 0.7 0.8 0.9 1 1 1 1 1 1
  spline S95 degree 5 poles (94.96, 44) (94.99, 44.0758) (95.05, 44.2209) (95.14, 44.4187) (95.26, 44.6419) (95.41, 44.8491) (95.56, 44.9779) (95.71, 45.022) (95.86, 44.9779) (96.01, 44.8491) (96.16, 44.6419) (96.28, 44.4187) (96.37, 44.2209) (96.43, 44.0758) (96.46, 44) knots 0 0 0 0 0 0 0.1 0.2 0.3 0.4 0.5 0.6 0.7 0.8 0.9 1 1 1 1 1 1
  line L21 (94.96, 44) -> (93, 5.4)
  line L22 (96.46, 44) -> (98.42, 5.4)
  line L23 (3, 5.4) -> (9, 5.4)
  line L24 (14.42, 5.4) -> (21, 5.4)
  line L25 (26.42, 5.4) -> (33, 5.4)
  line L26 (38.42, 5.4) -> (45, 5.4)
  line L27 (50.42, 5.4) -> (57, 5.4)
  line L28 (62.42, 5.4) -> (69, 5.4)
  line L29 (74.42, 5.4) -> (81, 5.4)
  line L30 (86.42, 5.4) -> (93, 5.4)
  line L31 (98.42, 5.4) -> (103, 5.4)
  line L32 (1.5, 44) -> (3, 5.4)
  line L33 (0, 44) -> (0, 0)
  spline S96 degree 5 poles (0, 44) (0.03, 44.0758) (0.09, 44.2209) (0.18, 44.4187) (0.3, 44.6419) (0.45, 44.8491) (0.6, 44.9779) (0.75, 45.022) (0.9, 44.9779) (1.05, 44.8491) (1.2, 44.6419) (1.32, 44.4187) (1.41, 44.2209) (1.47, 44.0758) (1.5, 44) knots 0 0 0 0 0 0 0.1 0.2 0.3 0.4 0.5 0.6 0.7 0.8 0.9 1 1 1 1 1 1
  line L34 (103.65, 44) -> (103, 5.4)
  line L35 (105.15, 44) -> (105.15, 0)
  spline S97 degree 5 poles (103.65, 44) (103.68, 44.0758) (103.74, 44.2209) (103.83, 44.4187) (103.95, 44.6419) (104.1, 44.8491) (104.25, 44.9779) (104.4, 45.022) (104.55, 44.9779) (104.7, 44.8491) (104.85, 44.6419) (104.97, 44.4187) (105.06, 44.2209) (105.12, 44.0758) (105.15, 44) knots 0 0 0 0 0 0 0.1 0.2 0.3 0.4 0.5 0.6 0.7 0.8 0.9 1 1 1 1 1 1
  point P0 (11.71, 45)
  point P1 (11.71, 45)
  point P2 (11.71, 45)
  point P3 (11.71, 45)
  point P4 (11.71, 45)
  point P5 (11.71, 45)
  point P6 (11.71, 45)
  point P7 (11.71, 45)
  point P8 (23.71, 45)
  point P9 (23.71, 45)
  point P10 (23.71, 45)
  point P11 (23.71, 45)
  point P12 (23.71, 45)
  point P13 (23.71, 45)
  point P14 (23.71, 45)
  point P15 (23.71, 45)
  point P16 (35.71, 45)
  point P17 (35.71, 45)
  point P18 (35.71, 45)
  point P19 (35.71, 45)
  point P20 (35.71, 45)
  point P21 (35.71, 45)
  point P22 (35.71, 45)
  point P23 (35.71, 45)
  point P24 (47.71, 45)
  point P25 (47.71, 45)
  point P26 (47.71, 45)
  point P27 (47.71, 45)
  point P28 (47.71, 45)
  point P29 (47.71, 45)
  point P30 (47.71, 45)
  point P31 (47.71, 45)
  point P32 (59.71, 45)
  point P33 (59.71, 45)
  point P34 (59.71, 45)
  point P35 (59.71, 45)
  point P36 (59.71, 45)
  point P37 (59.71, 45)
  point P38 (59.71, 45)
  point P39 (59.71, 45)
  point P40 (59.71, 45)
  point P41 (59.71, 45)
  point P42 (59.71, 45)
  point P43 (59.71, 45)
  point P44 (59.71, 45)
  point P45 (59.71, 45)
  point P46 (59.71, 45)
  point P47 (59.71, 45)
  point P48 (71.71, 45)
  point P49 (71.71, 45)
  point P50 (71.71, 45)
  point P51 (71.71, 45)
  point P52 (71.71, 45)
  point P53 (71.71, 45)
  point P54 (71.71, 45)
  point P55 (71.71, 45)
  point P56 (71.71, 45)
  point P57 (71.71, 45)
  point P58 (71.71, 45)
  point P59 (71.71, 45)
  point P60 (71.71, 45)
  point P61 (71.71, 45)
  point P62 (71.71, 45)
  point P63 (71.71, 45)
  point P64 (83.71, 45)
  point P65 (83.71, 45)
  point P66 (83.71, 45)
  point P67 (83.71, 45)
  point P68 (83.71, 45)
  point P69 (83.71, 45)
  point P70 (83.71, 45)
  point P71 (83.71, 45)
  point P72 (83.71, 45)
  point P73 (83.71, 45)
  point P74 (83.71, 45)
  point P75 (83.71, 45)
  point P76 (83.71, 45)
  point P77 (83.71, 45)
  point P78 (83.71, 45)
  point P79 (83.71, 45)
  point P80 (95.71, 45)
  point P81 (95.71, 45)
  point P82 (95.71, 45)
  point P83 (95.71, 45)
  point P84 (95.71, 45)
  point P85 (95.71, 45)
  point P86 (95.71, 45)
  point P87 (95.71, 45)
  point P88 (95.71, 45)
  point P89 (95.71, 45)
  point P90 (95.71, 45)
  point P91 (95.71, 45)
  point P92 (95.71, 45)
  point P93 (95.71, 45)
  point P94 (95.71, 45)
  point P95 (95.71, 45)
  point P96 (0.75, 45)
  point P97 (104.4, 45)
  constraint horizontal L0
  constraint coincident L0.start L33.end
  constraint horizontal L23
  constraint parallel L23 L24
  constraint parallel L24 L25
  constraint parallel L25 L26
  constraint parallel L26 L27
  constraint parallel L27 L28
  constraint parallel L28 L29
  constraint parallel L29 L30
  constraint parallel L0 L31
  constraint perpendicular L0 L33
  constraint perpendicular L0 L35
sketch "Sketch2" plane through (0, 0, 0) normal (0, 0, 1) x (1, 0, 0)
sketch "Sketch3" plane through (0, 0, 0) normal (0, 0, 1) x (1, 0, 0)
sketch "Sketch4" plane through (0, 0, 0) normal (0, 0, 1) x (1, 0, 0)
sketch "Sketch5" plane through (0, 0, 0) normal (0, 0, 1) x (1, 0, 0)
sketch "Sketch6" plane through (0, 0, 0) normal (0, 0, 1) x (1, 0, 0)
sketch "Sketch7" plane through (0, 0, 0) normal (0, 0, 1) x (1, 0, 0)
extrude "Extrude1" add sketch "Sketch1" against normal blind 180
sketch "Sketch8" plane through (0, 5.4, 0) normal (0, 1, 0) x (-1, 0, 0)
  line L0 (-3, 0) -> (-9, 0)
  line L1 (-9, 0) -> (-9, -180)
  line L2 (-9, -180) -> (-3, -180)
  line L3 (-3, -180) -> (-3, 0)
sketch "Sketch9" plane through (0, 5.4, 0) normal (0, 1, 0) x (-1, 0, 0)
  line L0 (-98.42, 0) -> (-103, 0)
  line L1 (-103, 0) -> (-103, -180)
  line L2 (-103, -180) -> (-98.42, -180)
  line L3 (-98.42, -180) -> (-98.42, 0)
sketch "Sketch10" plane through (0, 0, 0) normal (0, -1, 0) x (1, 0, 0)
  line L0 (105.15, 0) -> (0, 0)
  line L1 (0, 0) -> (0, -180)
  line L2 (0, -180) -> (105.15, -180)
  line L3 (105.15, -180) -> (105.15, 0)
  line L4 (18.492, -125, -45) -> (88.492, -125, -45)
  line L5 (88.492, -125, -45) -> (88.492, -55, -45)
  line L6 (88.492, -55, -45) -> (18.492, -55, -45)
  line L7 (18.492, -55, -45) -> (18.492, -125, -45)
